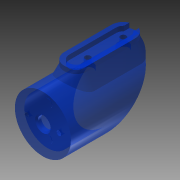
# Autodesk Inventor part: Motor Mount
Saved by Autodesk Inventor 2014 (Build 180170000, 170)
## iProperties
Created: 2014-02-04
Part Number: Motor Mount
Material: Glass
Document SubType Name: Modeling
Designer: Spooner
Density: 2.18 g/cm^3
Appearance: Clear - Blue
Mass: 25.079 g
Surface Area: 81.3813 cm^2
Volume: 11.5041 cm^3
Author: Spooner
Autodesk Inventor part; units mm, degrees
ref_plane "XZ Plane" through (0, 0, 0) normal (0, 1, 0) x (-1, 0, 0)
ref_plane "XY Plane" through (0, 0, 0) normal (0, 0, 1) x (1, 0, 0)
sketch "Sketch1" plane through (0, 0, 0) normal (0, 0, 1) x (1, 0, 0)
  circle A0 centre (0, 0) radius 12.5095
  circle A1 centre (0, 0) radius 3.429
  dimension "d0" = 25.019
  dimension "d1" = 6.858
  constraints: 2 centre point, 2 coincident
  measures "d0" diameter of A0
  measures "d1" diameter of A1
extrude "Extrusion1" add sketch "Sketch1" along normal blind 2.54
sketch "Sketch2" plane through (0, 0, 2.54) normal (0, 0, 1) x (1, 0, 0)
  circle A0 centre (0, 0) radius 3.429 projected
  point P0 (0, 8.5725)
  point P1 (0, -8.5725)
  dimension "d4" = 17.145
  dimension "d5" = 8.5725
  constraints: 2 vertical alignment
  measures "d4" distance of point (0, -8.572) point (0, 8.572)
  measures "d5" distance of point (0, -8.572) A0.centre
hole "Hole1" at (0, 8.5725, 2.54) at (0, -8.5725, 2.54) direction (0, 0, -1) diameter 2.4638 end through all
sketch "Sketch3" plane through (0, 0, 0) normal (0, 0, -1) x (-1, 0, 0)
  circle A0 centre (0, 0) radius 3.429 projected
  circle A1 centre (-8.3693, 0) radius 2.3495
  circle A2 centre (8.3693, 0) radius 2.3495
  dimension "d13" = 4.699
  dimension "d14" = 16.7386
  dimension "d15" = 8.3693
  constraints: 2 centre point, 2 horizontal alignment, 1 equal radius
  measures "d13" diameter of A1
  measures "d14" distance of A2.centre A1.centre
  measures "d15" distance of A0.centre A1.centre
extrude "Extrusion2" add sketch "Sketch3" along normal blind 0.508 contours A1 | A2
chamfer "Chamfer1" distance 0.381 angle 45 2 edges at (10.7188, 0, -0.508) (-6.0198, 0, -0.508)
chamfer "Chamfer2" distance 0.762 angle 45 1 edges at (-3.429, 0, 2.54)
sketch "Sketch4" plane through (0, 0, 2.54) normal (0, 0, 1) x (1, 0, 0)
  circle A0 centre (0, 0) radius 12.5095 projected
  circle A1 centre (0, 0) radius 4.191 projected
  circle A2 centre (0, 0) radius 15.0495
  dimension "d24" = 2.54
  constraints: 1 centre point, 1 coincident
  measures "d24" radial gap between concentric circles of A0 A2
extrude "Extrusion3" add sketch "Sketch4" against normal blind 18.9738 contours A2
ref_plane "Work Plane1" through (15.0495, 0, 2.54) normal (1, 0, 0) x (0, 1, 0)
ref_plane "Work Plane2" through (15.0495, 0, -16.4338) normal (0.7071068, 0, -0.7071068) x (0, 1, 0)
sketch "Sketch6" plane through (0, 0, -16.4338) normal (0, 0, -1) x (-1, 0, 0)
  circle A0 centre (0, 0) radius 12.5095 projected
  circle A1 centre (0, 0) radius 15.0495 projected
extrude "Extrusion4" add sketch "Sketch6" along normal up to surface surface through (15.0495, 0, -16.4338) normal (0.7071068, 0, -0.7071068)
ref_plane "Work Plane4" through (-18.8595, 0, 2.54) normal (1, 0, 0) x (0, 1, 0)
ref_plane "Work Plane3" through (-15.0495, 0, 2.54) normal (1, 0, 0) x (0, 1, 0)
sketch "Sketch7" plane through (-18.8595, 0, 2.54) normal (1, 0, 0) x (0, 1, 0)
  arc A0 (6.35, -17.78) -> (-6.35, -17.78) centre (0, -17.78) ccw
  arc A1 (-6.35, -43.18) -> (6.35, -43.18) centre (0, -43.18) ccw
  line L0 (6.35, -17.78) -> (6.35, -43.18)
  line L1 (-6.35, -17.78) -> (-6.35, -43.18)
  point P0 (0, -2.54)
  dimension "d31" = 25.4
  dimension "d32" = 12.7
  dimension "d33" = 15.24
  constraints: 4 end point, 4 point on circle, 4 tangent, 2 centre point, 2 vertical alignment, 1 equal radius
  measures "d31" distance of A1.centre A0.centre
  measures "d32" diameter of A0
  measures "d33" distance of A0.centre point (0, -2.54)
extrude "Extrusion5" add sketch "Sketch7" along normal up to surface draft 25 round surface about axis through (0, 0, 2.54) along (0, 0, -1) radius 15.0495 far side no
sketch "Sketch8" plane through (-18.8595, 0, 2.54) normal (-1, 0, 0) x (0, 0, 1)
  arc A0 (-17.78, -6.35) -> (-17.78, 6.35) centre (-17.78, 0) ccw projected
  line L0 (-43.18, 6.35) -> (-17.78, 6.35) projected
  arc A1 (-43.18, 6.35) -> (-43.18, -6.35) centre (-43.18, 0) ccw projected
  line L1 (-17.78, -6.35) -> (-43.18, -6.35) projected
  arc A2 (-17.78, -3.81) -> (-17.78, 3.81) centre (-17.78, 0) ccw
  line L2 (-17.78, -3.81) -> (-43.18, -3.81)
  arc A3 (-43.18, 3.81) -> (-43.18, -3.81) centre (-43.18, 0) ccw
  line L3 (-43.18, 3.81) -> (-17.78, 3.81)
  point P0 (-2.54, 0)
  dimension "d36" = 2.54
  constraints: 4 end point, 4 point on circle, 2 centre point, 3 other
  measures "d36" distance between parallel lines of L0 L3
extrude "Extrusion6" add sketch "Sketch8" along normal blind 2.54
sketch "Sketch9" plane through (-18.8595, 0, 2.54) normal (-1, 0, 0) x (0, 0, 1)
  arc A0 (-43.18, 3.81) -> (-43.18, -3.81) centre (-43.18, 0) ccw projected
  line L0 (-102.3269, 2.54) -> (-38.6775, 2.54)
  line L1 (-38.6775, 2.54) -> (-38.6775, -2.54)
  line L2 (-38.6775, -2.54) -> (-102.3269, -2.54)
  line L3 (-102.3269, -2.54) -> (-102.3269, 2.54)
  point P0 (-2.54, 0)
  point P1 (-38.6775, 0)
  dimension "d39" = 5.08
  constraints: 8 end point, 2 parallel, 1 horizontal, 1 horizontal alignment, 1 midpoint, 1 perpendicular
  measures "d39" distance of L0.end L1.end
extrude "Extrusion7" cut sketch "Sketch9" along normal blind 2.54
sketch "Sketch10" plane through (-18.8595, 0, 2.54) normal (-1, 0, 0) x (0, 0, 1)
  arc A0 (-46.0198, -2.54) -> (-43.18, -3.81) centre (-43.18, 0) ccw projected
  arc A1 (-17.78, -3.81) -> (-17.78, 3.81) centre (-17.78, 0) ccw projected
  circle A2 centre (-43.18, 0) radius 1.524
  circle A3 centre (-24.13, 0) radius 1.524
  point P0 (-2.54, 0)
  dimension "d42" = 19.05
  dimension "d43" = 3.048
  dimension "d44" = 6.35
  constraints: 2 centre point, 1 equal radius, 1 horizontal alignment
  measures "d42" distance of A2.centre A3.centre
  measures "d43" diameter of A3
  measures "d44" distance of A1.centre A3.centre
extrude "Extrusion8" cut sketch "Sketch10" against normal blind 12.7
sketch "Sketch11" plane through (-15.0495, 0, 2.54) normal (1, 0, 0) x (0, 1, 0)
  spline S0 degree 2 poles (0, -22.606) (2.6396, -22.606) (1.3198, -24.892) (0, -27.178) (-1.3198, -24.892) (-2.6396, -22.606) (0, -22.606) knots 0 0 0 0.333333 0.333333 0.666667 0.666667 1 1 1 weights 1 0.5 1 0.5 1 0.5 1 projected
  spline S1 degree 2 poles (0, -41.656) (2.6396, -41.656) (1.3198, -43.942) (0, -46.228) (-1.3198, -43.942) (-2.6396, -41.656) (0, -41.656) knots 0 0 0 0.333333 0.333333 0.666667 0.666667 1 1 1 weights 1 0.5 1 0.5 1 0.5 1 projected
  circle A0 centre (0, -24.13) radius 2.9464
  circle A1 centre (0, -43.18) radius 2.9464
  circle A2 centre (0, -24.13) radius 1.524 projected
  point P0 (0, -2.54)
  dimension "d47" = 5.8928
  constraints: 2 centre point, 1 equal radius, 1 horizontal alignment, 3 other
  measures "d47" diameter of A1
extrude "Extrusion9" cut sketch "Sketch11" along normal blind 12.7
sketch "Sketch12" plane through (15.0495, 0, -16.4338) normal (0.7071068, 0, -0.7071068) x (0, 1, 0)
  ellipse E0 centre (0, -21.2832) end of major axis (0, 0) minor radius 15.0495 (-9.1667, -38.1627) -> (9.1667, -38.1627) ccw projected
  line L0 (44.4371, -57.4729) -> (-31.8022, -57.4729)
  line L1 (-31.8022, -57.4729) -> (-31.8022, 17.7578)
  line L2 (-31.8022, 17.7578) -> (44.4371, 17.7578)
  line L3 (44.4371, 17.7578) -> (44.4371, -57.4729)
  point P0 (0, 0.9788)
  point P1 (-12.2564, -33.9332)
  point P2 (12.2564, -33.9332)
  point P3 (12.2564, -33.6337)
  point P4 (-12.2564, -33.6337)
  constraints: 8 end point, 2 parallel, 1 horizontal, 1 perpendicular, 2 other
extrude "Extrusion10" cut sketch "Sketch12" along normal through all
equation "\"d5\" = 0.5 * d4"
equation "\"d15\" = 0.5 * d14"
body "Solid1"
